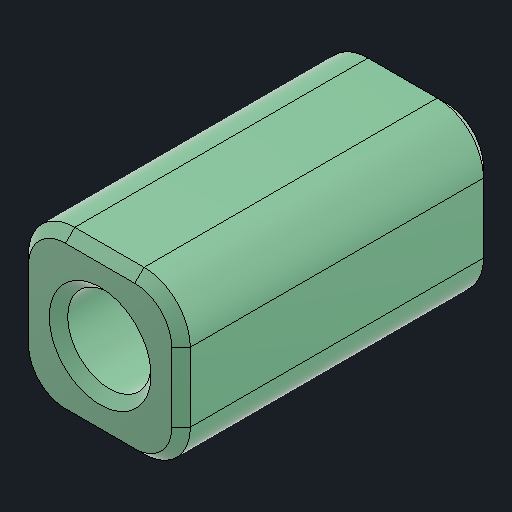
# Autodesk Inventor part: shaft-15mm-squareipt
Saved by Autodesk Inventor 2026 (Build 300175050, 175E)
## iProperties
Created: 2025-07-16
Part Number: shaft-15mm-squareipt
Material: ABS Plastic
Document SubType Name: Modeling
Designer: queezz
Density: 1.06 g/cm^3
Appearance: Smooth - Dark Sea Green
Author: queezz
Autodesk Inventor part; units mm, degrees
ref_plane "YZ Plane" through (0, 0, 0) normal (1, 0, 0) x (0, 1, 0)
ref_plane "XZ Plane" through (0, 0, 0) normal (0, 1, 0) x (-1, 0, 0)
ref_plane "XY Plane" through (0, 0, 0) normal (0, 0, 1) x (1, 0, 0)
sketch "Sketch1" plane through (0, 0, 0) normal (0, 0, 1) x (1, 0, 0)
  circle A0 centre (0, 0) radius 1.8
  line L0 (-3.5, 3.5) -> (3.5, 3.5)
  line L1 (3.5, 3.5) -> (3.5, -3.5)
  line L2 (3.5, -3.5) -> (-3.5, -3.5)
  line L3 (-3.5, -3.5) -> (-3.5, 3.5)
  point P0 (3.5, 0)
  point P1 (0, 3.5)
  dimension "d0" = 3.6
  dimension "d24" = 7
  constraints: 8 end point, 2 midpoint, 2 parallel, 2 perpendicular, 1 centre point, 1 coincident, 1 horizontal, 1 horizontal alignment, 1 vertical alignment
  measures "d0" diameter of A0
  measures "d24" distance of L0.start L0.end
extrude "Extrusion1" add sketch "Sketch1" along normal blind 13.5
fillet "Fillet3" radius 2 4 edges at (3.5, 3.5, 6.75) (3.5, -3.5, 6.75) (-3.5, -3.5, 6.75) (-3.5, 3.5, 6.75)
chamfer "Chamfer4" distance 0.4 angle 45 18 edges at (-2.9142, -2.9142, 13.5) (-3.5, 0, 13.5) (-2.9142, 2.9142, 13.5) (0, 3.5, 13.5) (2.9142, 2.9142, 13.5) (3.5, 0, 13.5) (2.9142, -2.9142, 13.5) (0, -3.5, 13.5) (2.9142, -2.9142, 0) (3.5, 0, 0) (2.9142, 2.9142, 0) (0, 3.5, 0) (-2.9142, 2.9142, 0) (-3.5, 0, 0) (-2.9142, -2.9142, 0) (0, -3.5, 0) (-1.8, 0, 13.5) (-1.8, 0, 0)
body "Solid1"
